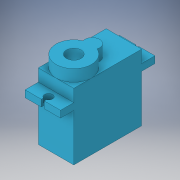
# Autodesk Inventor part: Servo body
Saved by Autodesk Inventor 2018 (Build 220112000, 112)
## iProperties
Created: 2018-06-25
Part Number: Servo body
Material: Generic
Document SubType Name: Modeling
Designer: Ajith Thomas
Density: 1 g/cm^3
Appearance: Turquoise
Mass: 6.65425 g
Surface Area: 27.8362 cm^2
Volume: 6.65425 cm^3
Author: Ajith Thomas
Autodesk Inventor part; units mm, degrees
ref_plane "YZ Plane" through (0, 0, 0) normal (1, 0, 0) x (0, 1, 0)
ref_plane "XZ Plane" through (0, 0, 0) normal (0, 1, 0) x (-1, 0, 0)
ref_plane "XY Plane" through (0, 0, 0) normal (0, 0, 1) x (1, 0, 0)
sketch "Sketch1" plane through (0, 0, 0) normal (0, 1, 0) x (-1, 0, 0)
  line L0 (6, 11.5) -> (-6, 11.5)
  line L1 (-6, 11.5) -> (-6, -11.5)
  line L2 (-6, -11.5) -> (6, -11.5)
  line L3 (6, -11.5) -> (6, 11.5)
  line L4 (6, 11.5) -> (-6, -11.5) construction
  line L5 (-6, 11.5) -> (6, -11.5) construction
  point P0 (0, 0)
  dimension "d0" = 12
  dimension "d1" = 23
  constraints: 12 end point, 2 midpoint, 2 parallel, 1 horizontal, 1 perpendicular
  measures "d0" distance of L2.end L1.end
  measures "d1" distance of L1.end L0.end
extrude "Extrusion1" add sketch "Sketch1" along normal mid plane 22.5
sketch "Sketch2" plane through (-6, 11.25, 11.5) normal (0, 0, 1) x (1, 0, 0)
  line L0 (12, -22.5) -> (0, -22.5) projected
  line L1 (0, -22.5) -> (0, 0) projected
  line L2 (0, -6.5) -> (12, -6.5)
  line L3 (12, -22.5) -> (12, 0) projected
  line L4 (0, -4.2) -> (12, -4.2)
  line L5 (0, -4.2) -> (0, -6.5)
  line L6 (12, -4.2) -> (12, -6.5)
  point P0 (6, -11.25)
  dimension "d4" = 16
  dimension "d5" = 2.3
  constraints: 8 end point, 4 point on line, 2 horizontal, 1 collinear, 1 perpendicular
  measures "d4" distance between parallel lines of L0 L2
  measures "d5" distance between parallel lines of L2 L4
extrude "Extrusion2" add sketch "Sketch2" along normal blind 4.5 contours L2 L1 L4 L3
mirror "Mirror1" about plane through (0, 0, 0) normal (0, 0, 1) of "Extrusion2"
sketch "Sketch3" plane through (-6, 7.05, 11.5) normal (0, 1, 0) x (1, 0, 0)
  arc A0 (6.5, -3.804) -> (5.5, -3.804) centre (6, -2.55) ccw
  line L0 (0, 0) -> (0, -4.5) projected
  line L1 (12, -4.5) -> (0, -4.5) construction
  line L2 (6, -2.55) -> (6, -4.5) construction
  line L3 (0, -4.5) -> (12, -4.5) construction
  line L4 (6, -2.55) -> (6, -1.2) construction
  line L5 (5.5, -4.5) -> (5.5, -3.804)
  line L6 (6.5, -4.5) -> (6.5, -3.804)
  line L7 (6.5, -4.5) -> (5.5, -4.5)
  point P0 (6, 11.5)
  point P1 (5.5, -2.8875)
  point P2 (6.5, -2.8875)
  dimension "d8" = 2.7
  dimension "d9" = 6
  dimension "d11" = 0.5
  dimension "d14" = 1.95
  constraints: 10 end point, 3 point on circle, 2 symmetric about line, 2 vertical, 1 centre point, 1 collinear, 1 midpoint, 1 point on line
  measures "d8" diameter of A0
  measures "d9" distance from line of L2.start L0
  measures "d11" distance between parallel lines of L5 L4
  measures "d14" distance from line of L1 L2.start
extrude "Extrusion3" cut sketch "Sketch3" against normal blind 4.5
mirror "Mirror2" about plane through (0, 0, 0) normal (0, 0, 1) of "Extrusion3"
sketch "Sketch4" plane through (0, 11.25, 0) normal (0, 1, 0) x (1, 0, 0)
  circle A0 centre (0, -5.5) radius 6
  line L0 (-6, 11.5) -> (-6, -11.5) projected
  line L1 (-6, -11.5) -> (6, -11.5) projected
  circle A1 centre (0, -5.5) radius 2.5
  point P0 (0, 0)
  dimension "d17" = 5
  constraints: 2 centre point, 2 tangent, 1 coincident
  measures "d17" diameter of A1
extrude "Extrusion4" add sketch "Sketch4" along normal blind 4 contours A0
sketch "Sketch5" plane through (0, 11.25, 0) normal (0, 1, 0) x (1, 0, 0)
  circle A0 centre (0, 0.75) radius 2.5
  circle A1 centre (0, -5.5) radius 2.5 projected
  point P0 (0, 0)
  dimension "d20" = 5
  dimension "d21" = 6.25
  constraints: 1 centre point
  measures "d20" diameter of A0
  measures "d21" distance of A1.centre A0.centre
extrude "Extrusion5" add sketch "Sketch5" along normal blind 4 contours A0
sketch "Sketch6" plane through (0, 11.25, 5.5) normal (0, 1, 0) x (1, 0, 0)
  circle A0 centre (0, 0) radius 2.5 projected
  point P0 (0, 5.5)
extrude "Extrusion6" cut sketch "Sketch6" against normal blind 10
body "Solid1"
